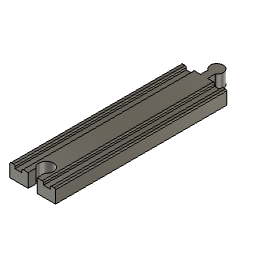
straight_train_track (Autodesk Fusion 360 design; units mm, degrees)
Autodesk Fusion 360 part; units mm, degrees
note: some values were not read from the file. Set by a fixed rule: which sketch regions a step uses.
sketch "Sketch1" plane through (0, 0, 0) normal (0, 0, 1) x (1, 0, 0)
  line L0 (0, 0) -> (40, 0)
  line L1 (40, 0) -> (40, 150)
  line L2 (40, 150) -> (0, 150)
  line L3 (0, 150) -> (0, 0)
  line L4 (17.1, 150) -> (23.3, 150)
  line L5 (23.3, 150) -> (23.3, 157)
  line L6 (23.3, 157) -> (17.1, 157)
  line L7 (17.1, 157) -> (17.1, 150)
  circle A0 centre (20.0369, 161.3) radius 5.7
  circle A1 centre (20, 11.85) radius 6.45
  line L8 (16.1, 0) -> (23.9, 0)
  line L9 (23.9, 0) -> (23.9, 7)
  line L10 (23.9, 7) -> (16.1, 7)
  line L11 (16.1, 7) -> (16.1, 0)
  dimension "d1" = 40
  dimension "d2" = 150
  dimension "d3" = 6.2
  dimension "d4" = 7
  dimension "d5" = 23.3
  dimension "d6" = 11.4
  dimension "d8" = 17
  dimension "d9" = 12.9
  dimension "d11" = 18.3
  dimension "d12" = 20
  dimension "d13" = 7.8
  dimension "d14" = 7
  dimension "d15" = 16.1
  constraint horizontal L0
  constraint vertical L1
  constraint horizontal L2
  constraint vertical L3
  constraint coincident L0.start L3.end
  constraint horizontal L4
  constraint vertical L5
  constraint horizontal L6
  constraint vertical L7
  constraint coincident L2 L4.start
  constraint horizontal L8
  constraint vertical L9
  constraint horizontal L10
  constraint vertical L11
  constraint coincident L0 L8.start
  measures "d1" distance of L0.start L0.end
  measures "d2" distance of L0.start L2.end
  measures "d3" distance of L4.start L4.end
  measures "d4" distance of L4.start L6.end
  measures "d5" distance of L2.end L5
  measures "d6" diameter of A0
  measures "d9" diameter of A1
  measures "d12" distance of L3 A1.centre
  measures "d13" distance of L8.start L8.end
  measures "d14" distance of L8.start L10.end
  measures "d15" distance of L3 L11
extrude "Extrude1" add sketch "Sketch1" along normal blind 12 contours L0 L1 L2 L3 L4 A1 L9 L11 | L2 L4 L5 L7 A0 | L5 L6 L7 A0 | L5 L6 L7 A0
sketch "Sketch2" plane through (0, 0, 12) normal (0, 0, 1) x (-1, 0, 0)
  line L0 (-23.9, 0) -> (-40, 0)
  line L1 (-40, 0) -> (-40, -150)
  line L2 (-40, -150) -> (-23.3, -150)
  line L3 (-23.3, -150) -> (-23.3, -156.6265)
  arc A0 (-23.3, -156.6265) -> (-17.1, -156.4148) centre (-20.0369, -161.3) ccw
  line L4 (-17.1, -156.4148) -> (-17.1, -150)
  line L5 (-17.1, -150) -> (0, -150)
  line L6 (0, -150) -> (0, 0)
  line L7 (0, 0) -> (-16.1, 0)
  line L8 (-16.1, 0) -> (-16.1, -6.7126)
  arc A1 (-23.9, -6.7126) -> (-16.1, -6.7126) centre (-20, -11.85) ccw
  line L9 (-23.9, -6.7126) -> (-23.9, 0)
  line L10 (-4.5, 0) -> (-10.5, 0)
  line L11 (-10.5, 0) -> (-10.5, -150)
  line L12 (-10.5, -150) -> (-4.5, -150)
  line L13 (-4.5, -150) -> (-4.5, 0)
  line L14 (-35.5, 0) -> (-29.5, 0)
  line L15 (-29.5, 0) -> (-29.5, -150)
  line L16 (-29.5, -150) -> (-35.5, -150)
  line L17 (-35.5, -150) -> (-35.5, 0)
  dimension "d18" = 6
  dimension "d19" = 150
  dimension "d20" = 4.5
  dimension "d21" = 6
  dimension "d22" = 150
  dimension "d23" = 4.5
  constraint horizontal L10
  constraint vertical L11
  constraint horizontal L12
  constraint vertical L13
  constraint coincident L7 L10.start
  constraint horizontal L14
  constraint vertical L15
  constraint horizontal L16
  constraint vertical L17
  constraint coincident L0 L14.start
  measures "d18" distance of L10.start L10.end
  measures "d19" distance of L10.start L12.end
  measures "d20" distance of L6 L13
  measures "d21" distance of L14.start L14.end
  measures "d22" distance of L14.start L16.end
  measures "d23" distance of L1 L17
extrude "Extrude2" cut sketch "Sketch2" against normal blind 2.9 contours L0 L2 L14 L15 L16 L17 | L5 L7 L10 L11 L12 L13
fillet "Fillet1" radius 1.1 6 edges at (4.5, 75, 12) (0, 75, 12) (10.5, 75, 12) (29.5, 75, 12) (35.5, 75, 12) (40, 75, 12)
